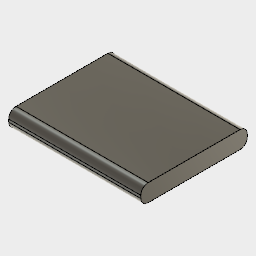
Wearable Camera Case (Autodesk Fusion 360 archive; units mm, degrees)
design "500mAh battery"
Autodesk Fusion 360 part; units mm, degrees
sketch "Sketch1" plane through (0, 0, 0) normal (0, 0, 1) x (1, 0, 0)
  line L0 (0, 0) -> (36, 0)
  line L1 (36, 0) -> (36, 29)
  line L2 (36, 29) -> (0, 29)
  line L3 (0, 29) -> (0, 0)
  dimension "d1" = 36
  dimension "d2" = 29
  constraint horizontal L0
  constraint vertical L1
  constraint horizontal L2
  constraint vertical L3
extrude "Extrude1" add sketch "Sketch1" along normal blind 4.75
fillet "Fillet1" radius 2 4 edges at (18, 0, 4.75) (18, 0, 0) (18, 29, 4.75) (18, 29, 0)

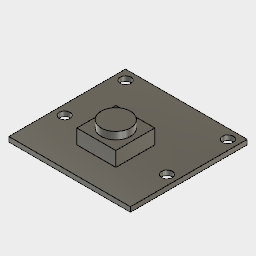
design "Pi Cam Module"
Autodesk Fusion 360 part; units mm, degrees
sketch "picam" plane through (0, 0, 0) normal (0, 0, 1) x (1, 0, 0)
  line L0 (0, 0) -> (25, 0)
  line L1 (25, 0) -> (25, -24)
  line L2 (25, -24) -> (0, -24)
  line L3 (0, -24) -> (0, 0)
  circle A0 centre (2, -2) radius 1.1
  line L4 (12.5, 0) -> (12.5, -24) construction
  circle A1 centre (2, -14.5) radius 1.1
  circle A2 centre (23, -2) radius 1.1
  circle A3 centre (23, -14.5) radius 1.1
  line L5 (16.5, -18.5) -> (8.5, -18.5)
  line L6 (8.5, -18.5) -> (8.5, -10.5)
  line L7 (8.5, -10.5) -> (16.5, -10.5)
  line L8 (16.5, -10.5) -> (16.5, -18.5)
  line L9 (16.5, -18.5) -> (8.5, -10.5) construction
  line L10 (8.5, -18.5) -> (16.5, -10.5) construction
  circle A4 centre (12.5, -14.5) radius 3
  dimension "d23" = 25
  dimension "d24" = 24
  dimension "d25" = 2.2
  dimension "d26" = 2
  dimension "d27" = 2
  dimension "d28" = 2.2
  dimension "d29" = 12.5
  dimension "d30" = 8
  dimension "d31" = 8
  dimension "d32" = 5.5
  dimension "d33" = 6
  constraint horizontal L0
  constraint vertical L1
  constraint horizontal L2
  constraint vertical L3
  constraint midpoint L0
  constraint midpoint L2
  constraint perpendicular L5 L6
  constraint parallel L5 L7
  constraint parallel L6 L8
  constraint horizontal L5
  constraint coincident L9
  constraint coincident L10
  constraint midpoint L10
  measures "d25" diameter of A0
  measures "d26" distance of L3
  measures "d27" distance of L0
  measures "d28" diameter of A1
  measures "d32" distance of L2 L5
  measures "d33" diameter of A4
extrude "Extrude6" add sketch "picam" against normal blind 1 contours L0 L1 L2 L3 | L5 L6 L7 L8 | A4
extrude "Extrude7" add sketch "picam" along normal blind 3 contours L5 L6 L7 L8 | A4
extrude "Extrude8" add sketch "picam" along normal blind 4.5 contours A4
equation "d38 = 3 mm + 1.5 mm"
named bodies: "picam"

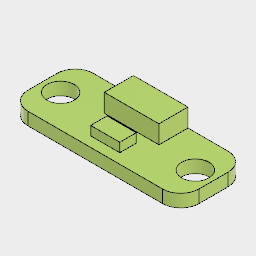
design "LED Sequin"
Autodesk Fusion 360 part; units mm, degrees
sketch "Sketch1" plane through (0, 0, 0) normal (0, 0, 1) x (1, 0, 0)
  line L0 (0, 0) -> (9.4, 0)
  line L1 (9.4, 0) -> (9.4, 3.6)
  line L2 (9.4, 3.6) -> (0, 3.6)
  line L3 (0, 3.6) -> (0, 0)
  line L4 (4.7, 3.6) -> (4.7, 0) construction
  line L5 (0, 1.8) -> (9.4, 1.8) construction
  line L6 (6.2, 2) -> (3.2, 2)
  line L7 (3.2, 2) -> (3.2, 3.6)
  line L8 (3.2, 3.6) -> (6.2, 3.6)
  line L9 (6.2, 3.6) -> (6.2, 2)
  line L10 (6.2, 2) -> (3.2, 3.6) construction
  line L11 (3.2, 2) -> (6.2, 3.6) construction
  circle A0 centre (1, 1.8) radius 0.75
  circle A1 centre (8.4, 1.8) radius 0.75
  line L12 (5.5, 0.5482) -> (3.9, 0.5482)
  line L13 (3.9, 0.5482) -> (3.9, 1.4482)
  line L14 (3.9, 1.4482) -> (5.5, 1.4482)
  line L15 (5.5, 1.4482) -> (5.5, 0.5482)
  line L16 (5.5, 0.5482) -> (3.9, 1.4482) construction
  line L17 (3.9, 0.5482) -> (5.5, 1.4482) construction
  dimension "d1" = 9.4
  dimension "d2" = 3.6
  dimension "d3" = 3
  dimension "d4" = 1.6
  dimension "d10" = 1.5
  dimension "d11" = 1
  dimension "d12" = 0.9
  dimension "d13" = 1.6
  constraint horizontal L0
  constraint vertical L1
  constraint horizontal L2
  constraint vertical L3
  constraint midpoint L2
  constraint midpoint L0
  constraint midpoint L3
  constraint midpoint L1
  constraint perpendicular L6 L7
  constraint parallel L6 L8
  constraint parallel L7 L9
  constraint horizontal L6
  constraint coincident L10
  constraint coincident L11
  constraint coincident L4
  constraint collinear L2 L8
  constraint coincident L5
  constraint perpendicular L12 L13
  constraint parallel L12 L14
  constraint parallel L13 L15
  constraint horizontal L12
  constraint coincident L16
  constraint coincident L17
  measures "d10" diameter of A0
  measures "d11" distance of L3
extrude "Extrude1" add sketch "Sketch1" against normal blind 0.7 contours L0 L1 L2 L3 L6 L7 L9 | L2 L6 L7 L8 L9 | L12 L13 L14 L15
extrude "Extrude2" add sketch "Sketch1" along normal blind 1 contours L2 L6 L7 L8 L9
fillet "Fillet1" radius 1 4 edges at (9.4, 3.6, -0.35) (0, 3.6, -0.35) (9.4, 0, -0.35) (0, 0, -0.35)
extrude "Extrude3" add sketch "Sketch1" along normal blind 0.5 contours L12 L13 L14 L15

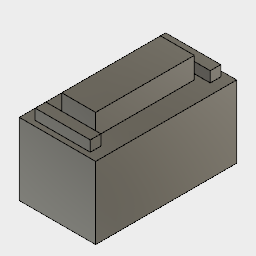
design "slim button"
Autodesk Fusion 360 part; units mm, degrees
sketch "Sketch1" plane through (0, 0, 0) normal (0, 0, 1) x (1, 0, 0)
  line L0 (0, 0) -> (3.6, 0)
  line L1 (3.6, 0) -> (3.6, 6.65)
  line L2 (3.6, 6.65) -> (0, 6.65)
  line L3 (0, 6.65) -> (0, 0)
  line L4 (0, 6.15) -> (3.6, 6.15) construction
  line L5 (3.1, 5.9) -> (0.5, 5.9)
  line L6 (0.5, 5.9) -> (0.5, 6.4)
  line L7 (0.5, 6.4) -> (3.1, 6.4)
  line L8 (3.1, 6.4) -> (3.1, 5.9)
  line L9 (3.1, 5.9) -> (0.5, 6.4) construction
  line L10 (0.5, 5.9) -> (3.1, 6.4) construction
  line L11 (1, 1) -> (2.6, 1)
  line L12 (2.6, 1) -> (2.6, 5.65)
  line L13 (2.6, 5.65) -> (1, 5.65)
  line L14 (1, 5.65) -> (1, 1)
  line L15 (0, 3.325) -> (3.6, 3.325) construction
  line L16 (0.5, 0.25) -> (3.1, 0.25)
  line L17 (0.5, 0.75) -> (0.5, 0.25)
  line L18 (3.1, 0.25) -> (3.1, 0.75)
  line L19 (3.1, 0.75) -> (0.5, 0.75)
  dimension "d1" = 3.6
  dimension "d2" = 6.65
  dimension "d3" = 1
  dimension "d10" = 0.5
  dimension "d11" = 0.5
  constraint horizontal L0
  constraint vertical L1
  constraint horizontal L2
  constraint vertical L3
  constraint coincident L3
  constraint coincident L1
  constraint perpendicular L1 L4
  constraint perpendicular L5 L6
  constraint parallel L5 L7
  constraint parallel L6 L8
  constraint horizontal L5
  constraint coincident L9
  constraint coincident L10
  constraint midpoint L4
  constraint midpoint L3
  constraint midpoint L1
  measures "d3" distance of L0
  measures "d10" distance of L2 L4
extrude "Extrude1" add sketch "Sketch1" against normal blind 3.4 contours L0 L1 L2 L3 | L5 L6 L7 L8 | L11 L12 L13 L14 | L16 L17 L18 L19
extrude "Extrude3" add sketch "Sketch1" along normal blind 1 contours L11 L12 L13 L14
extrude "Extrude4" add sketch "Sketch1" along normal blind 0.5 contours L5 L6 L7 L8 | L16 L17 L18 L19

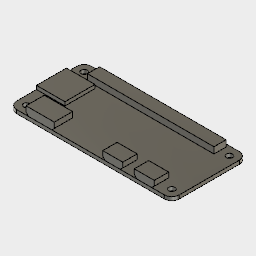
design "RaspPi Zero"
Autodesk Fusion 360 part; units mm, degrees
sketch "Sketch1" plane through (0, 0, 0) normal (0, 0, 1) x (1, 0, 0)
  line L0 (0, 0) -> (65, 0)
  line L1 (65, 0) -> (65, 30)
  line L2 (65, 30) -> (0, 30)
  line L3 (0, 30) -> (0, 0)
  circle A0 centre (3.5, 26.5) radius 1.25
  line L4 (32.5, 30) -> (32.5, 0) construction
  line L5 (0, 15) -> (65, 15) construction
  circle A1 centre (61.5, 26.5) radius 1.25
  circle A2 centre (3.5, 3.5) radius 1.25
  circle A3 centre (61.5, 3.5) radius 1.25
  line L6 (0, 22.9) -> (11.4, 22.9)
  line L7 (11.4, 22.9) -> (11.4, 10.9)
  line L8 (11.4, 10.9) -> (0, 10.9)
  line L9 (0, 10.9) -> (0, 22.9)
  line L10 (0, 16.9) -> (11.4, 16.9) construction
  line L11 (6.75, 7.3) -> (18.05, 7.3)
  line L12 (18.05, 7.3) -> (18.05, 0)
  line L13 (18.05, 0) -> (6.75, 0)
  line L14 (6.75, 0) -> (6.75, 7.3)
  line L15 (12.4, 7.3) -> (12.4, 0) construction
  line L16 (37.4, 5.75) -> (45.4, 5.75)
  line L17 (45.4, 5.75) -> (45.4, 0)
  line L18 (45.4, 0) -> (37.4, 0)
  line L19 (37.4, 0) -> (37.4, 5.75)
  line L20 (41.4, 5.75) -> (41.4, 0) construction
  line L21 (50, 5.75) -> (58, 5.75)
  line L22 (58, 5.75) -> (58, 0)
  line L23 (58, 0) -> (50, 0)
  line L24 (50, 0) -> (50, 5.75)
  line L25 (54, 5.75) -> (54, 0) construction
  line L26 (57.77, 24.05) -> (7.23, 24.05)
  line L27 (7.23, 24.05) -> (7.23, 28.95)
  line L28 (7.23, 28.95) -> (57.77, 28.95)
  line L29 (57.77, 28.95) -> (57.77, 24.05)
  line L30 (57.77, 24.05) -> (7.23, 28.95) construction
  line L31 (7.23, 24.05) -> (57.77, 28.95) construction
  dimension "d1" = 65
  dimension "d2" = 30
  dimension "d3" = 2.5
  dimension "d4" = 3.5
  dimension "d5" = 3.5
  dimension "d6" = 12
  dimension "d7" = 11.4
  dimension "d8" = 16.9
  dimension "d9" = 11.3
  dimension "d10" = 7.3
  dimension "d11" = 12.4
  dimension "d12" = 8
  dimension "d13" = 5.75
  dimension "d14" = 41.4
  dimension "d15" = 8
  dimension "d16" = 5.75
  dimension "d17" = 54
  dimension "d28" = 50.54
  dimension "d29" = 4.9
  dimension "d30" = 3.5
  constraint horizontal L0
  constraint vertical L1
  constraint horizontal L2
  constraint vertical L3
  constraint midpoint L2
  constraint midpoint L0
  constraint midpoint L3
  constraint midpoint L1
  constraint horizontal L6
  constraint vertical L7
  constraint horizontal L8
  constraint vertical L9
  constraint midpoint L9
  constraint midpoint L7
  constraint collinear L3 L9
  constraint horizontal L11
  constraint vertical L12
  constraint horizontal L13
  constraint vertical L14
  constraint midpoint L11
  constraint midpoint L13
  constraint collinear L0 L13
  constraint horizontal L16
  constraint vertical L17
  constraint horizontal L18
  constraint vertical L19
  constraint midpoint L16
  constraint midpoint L18
  constraint collinear L0 L18
  constraint horizontal L21
  constraint vertical L22
  constraint horizontal L23
  constraint vertical L24
  constraint midpoint L21
  constraint midpoint L23
  constraint collinear L0 L23
  constraint perpendicular L26 L27
  constraint parallel L26 L28
  constraint parallel L27 L29
  constraint horizontal L26
  constraint coincident L30
  constraint coincident L31
  constraint coincident L4
  measures "d3" diameter of A0
  measures "d4" distance of L3
  measures "d5" distance of L2
  measures "d8" distance of L0 L10
  measures "d11" distance of L3 L15
  measures "d14" distance of L3 L20
  measures "d17" distance of L3 L25
  measures "d30" distance of L2
extrude "Extrude1" add sketch "Sketch1" against normal blind 1.45 contours L0 L1 L2 L3 L6 L7 L8 L11 L12 L14 L16 L17 L19 L21 L22 L24 | L0 L11 L12 L13 L14 | L3 L6 L7 L8 L9 | L0 L16 L17 L18 L19 | L0 L21 L22 L23 L24 | L26 L27 L28 L29 makes body 1
fillet "Fillet1" radius 3 4 edges at (0, 0, -0.725) (0, 30, -0.725) (65, 30, -0.725) (65, 0, -0.725) on bodies 1
extrude "Extrude2" add sketch "Sketch1" along normal blind 1.45 separate body contours L3 L6 L7 L8 L9 makes body 2
extrude "Extrude3" add sketch "Sketch1" along normal blind 3.19 separate body contours L0 L11 L12 L13 L14 makes body 3
extrude "Extrude4" add sketch "Sketch1" along normal blind 3 separate body contours L0 L16 L17 L18 L19 | L0 L21 L22 L23 L24 makes body 4 at (42.7333, 1.9167, 0) makes body 5 at (52.6667, 3.8333, 0)
chamfer "Chamfer1" distance 1 angle 45 6 edges at (50, 2.875, 0) (58, 2.875, 0) (6.75, 3.65, 0) (18.05, 3.65, 0) (37.4, 2.875, 0) (45.4, 2.875, 0) on bodies 3 4 5
extrude "Extrude5" add sketch "Sketch1" along normal blind 2.5 contours L26 L27 L28 L29 bodies 1

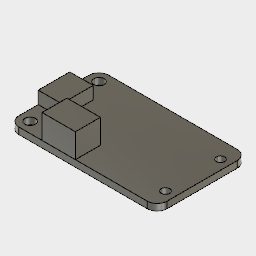
design "Powerboost 500C"
Autodesk Fusion 360 part; units mm, degrees
sketch "Sketch1" plane through (0, 0, 0) normal (0, 0, 1) x (1, 0, 0)
  line L0 (0, 0) -> (35.56, 0)
  line L1 (35.56, 0) -> (35.56, 21.59)
  line L2 (35.56, 21.59) -> (0, 21.59)
  line L3 (0, 21.59) -> (0, 0)
  circle A0 centre (2.54, 2.54) radius 1.25
  circle A1 centre (2.5519, 19.05) radius 1.25
  line L4 (15.94, 0) -> (7.94, 0)
  line L5 (7.94, 0) -> (7.94, 6)
  line L6 (7.94, 6) -> (15.94, 6)
  line L7 (15.94, 6) -> (15.94, 0)
  line L8 (15.94, 0) -> (7.94, 6) construction
  line L9 (7.94, 0) -> (15.94, 6) construction
  line L10 (5.65, 6.99) -> (0, 6.99)
  line L11 (0, 6.99) -> (0, 14.59)
  line L12 (0, 14.59) -> (5.65, 14.59)
  line L13 (5.65, 14.59) -> (5.65, 6.99)
  line L14 (5.65, 6.99) -> (0, 14.59) construction
  line L15 (0, 6.99) -> (5.65, 14.59) construction
  circle A2 centre (33.27, 17.51) radius 1
  line L16 (35.56, 10.795) -> (20, 10.795) construction
  circle A3 centre (33.27, 4.3) radius 1
  dimension "d1" = 35.56
  dimension "d2" = 21.59
  dimension "d3" = 2.5
  dimension "d4" = 2.54
  dimension "d5" = 2.54
  dimension "d6" = 2.5
  dimension "d9" = 8
  dimension "d10" = 6
  dimension "d11" = 11.94
  dimension "d13" = 5.65
  dimension "d14" = 7.6
  dimension "d16" = 2
  dimension "d46" = 16.51
  dimension "d47" = 2
  dimension "d49" = 13.21
  dimension "d51" = 33.27
  dimension "d52" = 33.27
  dimension "d53" = 4.3
  dimension "d61" = 10.8
  constraint horizontal L0
  constraint vertical L1
  constraint horizontal L2
  constraint vertical L3
  constraint perpendicular L4 L5
  constraint parallel L4 L6
  constraint parallel L5 L7
  constraint horizontal L4
  constraint coincident L8
  constraint coincident L9
  constraint perpendicular L10 L11
  constraint parallel L10 L12
  constraint parallel L11 L13
  constraint horizontal L10
  constraint coincident L14
  constraint coincident L15
  constraint collinear L3 L11
  constraint midpoint L1
  constraint perpendicular L1 L16
  constraint collinear L0 L4
  measures "d3" diameter of A0
  measures "d4" distance of L0
  measures "d5" distance of L3
  measures "d6" diameter of A1
  measures "d11" distance of L3
  measures "d16" diameter of A2
  measures "d47" diameter of A3
  measures "d51" distance of L3
  measures "d52" distance of L3
  measures "d53" distance of L0
  measures "d61" distance of L2
extrude "Extrude1" add sketch "Sketch1" against normal blind 1.6 makes body 1
fillet "Fillet1" radius 2.36 4 edges at (0, 0, -0.8) (0, 21.59, -0.8) (35.56, 21.59, -0.8) (35.56, 0, -0.8) on bodies 1
extrude "Extrude2" add sketch "Sketch1" along normal blind 3 separate body contours L3 L10 L11 L12 L13 makes body 2
extrude "Extrude3" add sketch "Sketch1" along normal blind 5.8 separate body contours L0 L4 L5 L6 L7 makes body 3
sketch "Sketch3" plane through (0, 0, -1.6) normal (0, 0, -1) x (1, 0, 0)
  arc A0 (35.56, -2.36) -> (33.2, 0) centre (33.2, -2.36) ccw construction
  line L0 (33.2, 0) -> (2.36, 0) construction
  arc A1 (2.36, 0) -> (0, -2.36) centre (2.36, -2.36) ccw construction
  line L1 (0, -2.36) -> (0, -19.23) construction
  arc A2 (0, -19.23) -> (2.36, -21.59) centre (2.36, -19.23) ccw construction
  line L2 (2.36, -21.59) -> (33.2, -21.59) construction
  arc A3 (33.2, -21.59) -> (35.56, -19.23) centre (33.2, -19.23) ccw construction
  line L3 (35.56, -19.23) -> (35.56, -2.36) construction
  circle A4 centre (2.5519, -19.05) radius 1.25
  circle A5 centre (33.27, -4.3) radius 1
  circle A6 centre (33.27, -17.51) radius 1
  circle A7 centre (2.54, -2.54) radius 1.25
  circle A8 centre (2.54, -2.54) radius 3
  circle A9 centre (2.5519, -19.05) radius 3
  circle A10 centre (33.27, -4.3) radius 3
  circle A11 centre (33.27, -17.51) radius 3
  line L4 (17.78, 0) -> (17.78, -21.59) construction
  line L5 (0, -10.795) -> (35.56, -10.795) construction
  line L6 (28, -17) -> (7.56, -17)
  line L7 (7.56, -17) -> (7.56, -4.59)
  line L8 (7.56, -4.59) -> (28, -4.59)
  line L9 (28, -4.59) -> (28, -17)
  line L10 (28, -17) -> (7.56, -4.59) construction
  line L11 (7.56, -17) -> (28, -4.59) construction
  line L12 (-1, -2.36) -> (-1, -19.23)
  arc A12 (-1, -19.23) -> (2.36, -22.59) centre (2.36, -19.23) ccw
  line L13 (2.36, -22.59) -> (33.2, -22.59)
  arc A13 (33.2, -22.59) -> (36.56, -19.23) centre (33.2, -19.23) ccw
  line L14 (36.56, -19.23) -> (36.56, -2.36)
  arc A14 (36.56, -2.36) -> (33.2, 1) centre (33.2, -2.36) ccw
  line L15 (33.2, 1) -> (2.36, 1)
  arc A15 (2.36, 1) -> (-1, -2.36) centre (2.36, -2.36) ccw
  dimension "d62" = 6
  dimension "d63" = 6
  dimension "d64" = 6
  dimension "d65" = 6
  dimension "d66" = 1
  constraint concentric A7 A8
  constraint concentric A4 A9
  constraint concentric A5 A10
  constraint concentric A6 A11
  constraint midpoint L0
  constraint midpoint L2
  constraint midpoint L1
  constraint midpoint L3
  constraint perpendicular L6 L7
  constraint parallel L6 L8
  constraint parallel L7 L9
  constraint horizontal L6
  constraint coincident L10
  constraint coincident L11
  constraint midpoint L4
  measures "d62" diameter of A8
  measures "d63" diameter of A9
  measures "d64" diameter of A10
  measures "d65" diameter of A11
  measures "d66" distance of L1
extrude "Extrude11" [rolled back] along distance 4 against distance -3 taper angle 0
extrude "Extrude12" [rolled back] along distance 3 taper angle 0
extrude "Extrude13" [rolled back] along distance -2 taper angle 0

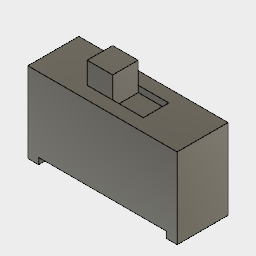
design "slide switch"
Autodesk Fusion 360 part; units mm, degrees
sketch "Sketch1" plane through (0, 0, 0) normal (0, 0, 1) x (1, 0, 0)
  line L0 (0, 0) -> (11.7, 0)
  line L1 (11.7, 0) -> (11.7, -4)
  line L2 (11.7, -4) -> (0, -4)
  line L3 (0, -4) -> (0, 0)
  line L4 (5.85, 0) -> (5.85, -4) construction
  line L5 (0, -2) -> (11.7, -2) construction
  line L6 (8.05, -3) -> (3.65, -3)
  line L7 (3.65, -3) -> (3.65, -1)
  line L8 (3.65, -1) -> (8.05, -1)
  line L9 (8.05, -1) -> (8.05, -3)
  line L10 (8.05, -3) -> (3.65, -1) construction
  line L11 (3.65, -3) -> (8.05, -1) construction
  line L12 (3.65, -1) -> (5.65, -1)
  line L13 (5.65, -1) -> (5.65, -3)
  line L14 (5.65, -3) -> (3.65, -3)
  line L15 (3.65, -3) -> (3.65, -1)
  dimension "d1" = 11.7
  dimension "d2" = 4
  dimension "d3" = 4.4
  dimension "d4" = 2
  dimension "d5" = 2
  constraint horizontal L0
  constraint vertical L1
  constraint horizontal L2
  constraint vertical L3
  constraint midpoint L0
  constraint midpoint L2
  constraint midpoint L3
  constraint midpoint L1
  constraint perpendicular L6 L7
  constraint parallel L6 L8
  constraint parallel L7 L9
  constraint horizontal L6
  constraint coincident L10
  constraint coincident L11
  constraint midpoint L5
  constraint horizontal L12
  constraint vertical L13
  constraint horizontal L14
extrude "Extrude1" add sketch "Sketch1" against normal blind 6.3 contours L0 L1 L2 L3 | L6 L8 L9 L13 | L6 L7 L8 L12 L13 L14 L15
extrude "Extrude2" cut sketch "Sketch1" against normal blind 0.5 contours L6 L8 L9 L13 | L6 L7 L8 L12 L13 L14 L15
extrude "Extrude3" add sketch "Sketch1" along normal blind 1.7 and the other way blind 0.5 contours L6 L7 L8 L12 L13 L14 L15
sketch "Sketch2" plane through (0, 0, -6.3) normal (0, 0, -1) x (1, 0, 0)
  line L0 (11.7, 4) -> (0, 4)
  line L1 (0, 4) -> (0, 0)
  line L2 (0, 0) -> (11.7, 0)
  line L3 (11.7, 0) -> (11.7, 4)
  line L4 (5.85, 4) -> (5.85, 0) construction
  line L5 (0, 2) -> (11.7, 2) construction
  line L6 (10.85, 0) -> (0.85, 0)
  line L7 (0.85, 0) -> (0.85, 4)
  line L8 (0.85, 4) -> (10.85, 4)
  line L9 (10.85, 4) -> (10.85, 0)
  line L10 (10.85, 0) -> (0.85, 4) construction
  line L11 (0.85, 0) -> (10.85, 4) construction
  dimension "d13" = 10
  dimension "d14" = 4
  constraint midpoint L0
  constraint midpoint L2
  constraint midpoint L1
  constraint midpoint L3
  constraint perpendicular L6 L7
  constraint parallel L6 L8
  constraint parallel L7 L9
  constraint horizontal L6
  constraint coincident L10
  constraint coincident L11
  constraint midpoint L4
extrude "Extrude4" cut sketch "Sketch2" against normal blind 0.5 contours L0 L2 L6 L7 L8 L9
